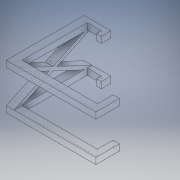
# Autodesk Inventor part: StrumClip1
Saved by Autodesk Inventor 2017 (Build 210142000, 142)
## iProperties
Created: 2017-12-03
Part Number: StrumClip1
Material: Generic
Document SubType Name: Modeling
Designer: Max
Density: 1 g/cm^3
Appearance: Default
Author: Max
Autodesk Inventor part; units mm, degrees
ref_plane "YZ Plane" through (0, 0, 0) normal (1, 0, 0) x (0, 1, 0)
ref_plane "XZ Plane" through (0, 0, 0) normal (0, 1, 0) x (-1, 0, 0)
ref_plane "XY Plane" through (0, 0, 0) normal (0, 0, 1) x (1, 0, 0)
sketch "Sketch1" plane through (0, 0, 0) normal (0, 0, 1) x (1, 0, 0)
  line L0 (0, 0) -> (0, 41.5)
  line L1 (0, 41.5) -> (9, 41.5)
  line L2 (12, 44.5) -> (8, 44.5)
  line L3 (9, 38.5) -> (12, 38.5)
  line L4 (12, 38.5) -> (12, 44.5)
  line L5 (8, 44.5) -> (-5, 44.5)
  line L6 (-5, 44.5) -> (-5, -5)
  line L7 (-5, -5) -> (52, -5)
  line L8 (9, 41.5) -> (9, 38.5)
  line L9 (48, 0) -> (48, 10)
  line L10 (48, 10) -> (52, 10)
  line L11 (48, 0) -> (0, 0)
  line L12 (52, 10) -> (52, -5)
  dimension "d0" = 41.5
  dimension "d2" = 3
  dimension "d7" = 5
  dimension "d8" = 3
  dimension "d9" = 9
  dimension "d10" = 3
  dimension "d20" = 10
  dimension "d22" = 5
  dimension "d23" = 4
  dimension "d24" = 48
  constraints: 26 end point, 4 perpendicular, 4 vertical, 2 horizontal, 2 parallel
  measures "d0" distance of L0.start L0.end
  measures "d2" distance of L3.end L3.start
  measures "d7" distance between parallel lines of L6 L0
  measures "d8" distance between parallel lines of L3 L1
  measures "d9" distance of L0.end L1.end
  measures "d10" distance between parallel lines of L5 L1
  measures "d20" distance of L9.start L9.end
  measures "d22" distance between parallel lines of L7 L11
  measures "d23" distance of L9.end L10.end
  measures "d24" distance between parallel lines of L0 L9
extrude "Extrusion1" add sketch "Sketch1" along normal blind 4
pattern_linear "Rectangular Pattern1" count 2 spacing 25 along (0, 0, 1) of "Extrusion1"
sketch "Sketch2" plane through (0, 0, 4) normal (0, 0, 1) x (1, 0, 0)
  line L0 (-5, 44.5) -> (-5, -5) projected
  line L1 (-5, -5) -> (0, -5)
  line L2 (0, -5) -> (0, 0)
  line L3 (0, 0) -> (-5, 0)
  line L4 (-5, 0) -> (-5, -5)
  constraints: 8 end point, 2 parallel, 1 horizontal, 1 perpendicular
sketch "Sketch3" plane through (0, 0, 25) normal (1, 0, 0) x (0, 0, -1)
  line L0 (25, 0) -> (21, 0) projected
  line L1 (21, 0) -> (0, 44.5)
  constraints: 2 end point
sweep "Sweep1" add profiles "Sketch2" path "Sketch3" keep normal constant yes
sketch "Sketch4" plane through (52, -5, 25) normal (0, 0, -1) x (-1, 0, 0)
  line L0 (52, 5) -> (52, 0) projected
  line L1 (57, 0) -> (0, 0) projected
  line L2 (52, 5) -> (57, 5)
  line L3 (57, 5) -> (57, 0)
  line L4 (57, 0) -> (52, 0)
  line L5 (52, 0) -> (52, 5)
  constraints: 8 end point, 2 parallel, 1 horizontal, 1 perpendicular
sketch "Sketch5" plane through (-5, -5, 0) normal (-1, 0, 0) x (0, 0, 1)
  line L0 (4, 49.5) -> (25, 5)
  point P0 (0, 5)
  constraints: 2 end point
sweep "Sweep2" add profiles "Sketch4" path "Sketch5"
body "Solid1"
